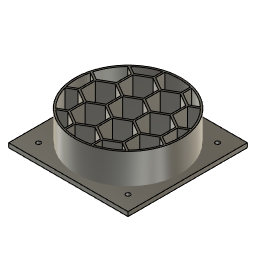
Wind Sim v6 (Autodesk Fusion 360 design; units mm, degrees)
Autodesk Fusion 360 part; units mm, degrees
(part 1 of 3)
sketch "Sketch3" plane through (0, 0, 0) normal (0, 0, 1) x (1, 0, 0)
  line L0 (-70.0229, 69.922) -> (69.9771, 69.922)
  line L1 (69.9771, 69.922) -> (69.9771, -70.078)
  line L2 (69.9771, -70.078) -> (-70.0229, -70.078)
  line L3 (-70.0229, -70.078) -> (-70.0229, 69.922)
  circle A0 centre (0, 0) radius 60
  line L4 (15, 8.6603) -> (0, 17.3205)
  line L5 (0, 17.3205) -> (-15, 8.6603)
  line L6 (-15, 8.6603) -> (-15, -8.6603)
  line L7 (-15, -8.6603) -> (0, -17.3205)
  line L8 (0, -17.3205) -> (15, -8.6603)
  line L9 (15, -8.6603) -> (15, 8.6603)
  line L10 (-15, 8.6603) -> (-15, -8.6603)
  line L11 (15, -8.6603) -> (15, 8.6603)
  line L12 (0, 17.3205) -> (-15, 8.6603)
  line L13 (15, 8.6603) -> (0, 17.3205)
  line L14 (17, 8.6603) -> (17, -8.6603)
  line L15 (17, -8.6603) -> (32, -17.3205)
  line L16 (47, -8.6603) -> (47, 8.6603)
  line L17 (47, -8.6603) -> (47, 8.6603)
  line L18 (17, 8.6603) -> (17, -8.6603)
  line L19 (47, 8.6603) -> (32, 17.3205)
  line L20 (32, -17.3205) -> (47, -8.6603)
  line L21 (32, 17.3205) -> (17, 8.6603)
  line L22 (32, 17.3205) -> (17, 8.6603)
  line L23 (47, 8.6603) -> (32, 17.3205)
  line L24 (-32, -17.3205) -> (-17, -8.6603)
  line L25 (-32, 17.3205) -> (-47, 8.6603)
  line L26 (-32, 17.3205) -> (-47, 8.6603)
  line L27 (-17, 8.6603) -> (-32, 17.3205)
  line L28 (-47, -8.6603) -> (-32, -17.3205)
  line L29 (-17, 8.6603) -> (-32, 17.3205)
  line L30 (-17, -8.6603) -> (-17, 8.6603)
  line L31 (-47, 8.6603) -> (-47, -8.6603)
  line L32 (-17, -8.6603) -> (-17, 8.6603)
  line L33 (-47, 8.6603) -> (-47, -8.6603)
  line L34 (-49, -8.6603) -> (-49, 8.6603)
  line L35 (-49, -8.6603) -> (-49, 8.6603)
  line L36 (-64, -17.3205) -> (-49, -8.6603)
  line L37 (-79, 8.6603) -> (-79, -8.6603)
  line L38 (-79, 8.6603) -> (-79, -8.6603)
  line L39 (-49, 8.6603) -> (-64, 17.3205)
  line L40 (-79, -8.6603) -> (-64, -17.3205)
  line L41 (-64, 17.3205) -> (-79, 8.6603)
  line L42 (-49, 8.6603) -> (-64, 17.3205)
  line L43 (-64, 17.3205) -> (-79, 8.6603)
  line L44 (79, -8.6603) -> (79, 8.6603)
  line L45 (49, 8.6603) -> (49, -8.6603)
  line L46 (49, 8.6603) -> (49, -8.6603)
  line L47 (79, -8.6603) -> (79, 8.6603)
  line L48 (49, -8.6603) -> (64, -17.3205)
  line L49 (64, 17.3205) -> (49, 8.6603)
  line L50 (79, 8.6603) -> (64, 17.3205)
  line L51 (64, -17.3205) -> (79, -8.6603)
  line L52 (64, 17.3205) -> (49, 8.6603)
  line L53 (79, 8.6603) -> (64, 17.3205)
  line L54 (-31, -19.3397) -> (-31, -36.6603)
  line L55 (-31, -19.3397) -> (-31, -36.6603)
  line L56 (-1, -36.6603) -> (-1, -19.3397)
  line L57 (-1, -36.6603) -> (-1, -19.3397)
  line L58 (-1, -19.3397) -> (-16, -10.6795)
  line L59 (-31, -36.6603) -> (-16, -45.3205)
  line L60 (-16, -10.6795) -> (-31, -19.3397)
  line L61 (-16, -10.6795) -> (-31, -19.3397)
  line L62 (-1, -19.3397) -> (-16, -10.6795)
  line L63 (-16, -45.3205) -> (-1, -36.6603)
  line L64 (-1, -36.6603) -> (-1, -19.3397)
  line L65 (-31, -36.6603) -> (-16, -45.3205)
  line L66 (-1, -19.3397) -> (-16, -10.6795)
  line L67 (-1, -36.6603) -> (-1, -19.3397)
  line L68 (-31, -19.3397) -> (-31, -36.6603)
  line L69 (-31, -19.3397) -> (-31, -36.6603)
  line L70 (-16, -10.6795) -> (-31, -19.3397)
  line L71 (-16, -45.3205) -> (-1, -36.6603)
  line L72 (-16, -10.6795) -> (-31, -19.3397)
  line L73 (-1, -19.3397) -> (-16, -10.6795)
  line L74 (16, -45.3205) -> (31, -36.6603)
  line L75 (31, -36.6603) -> (31, -19.3397)
  line L76 (31, -19.3397) -> (16, -10.6795)
  line L77 (16, -45.3205) -> (31, -36.6603)
  line L78 (31, -19.3397) -> (16, -10.6795)
  line L79 (1, -19.3397) -> (1, -36.6603)
  line L80 (16, -10.6795) -> (1, -19.3397)
  line L81 (1, -36.6603) -> (16, -45.3205)
  line L82 (1, -19.3397) -> (1, -36.6603)
  line L83 (1, -19.3397) -> (1, -36.6603)
  line L84 (16, -10.6795) -> (1, -19.3397)
  line L85 (31, -36.6603) -> (31, -19.3397)
  line L86 (31, -36.6603) -> (31, -19.3397)
  line L87 (16, -10.6795) -> (1, -19.3397)
  line L88 (1, -19.3397) -> (1, -36.6603)
  line L89 (31, -19.3397) -> (16, -10.6795)
  line L90 (31, -19.3397) -> (16, -10.6795)
  line L91 (31, -36.6603) -> (31, -19.3397)
  line L92 (1, -36.6603) -> (16, -45.3205)
  line L93 (16, -10.6795) -> (1, -19.3397)
  line L94 (-48, -10.6795) -> (-63, -19.3397)
  line L95 (-63, -36.6603) -> (-48, -45.3205)
  line L96 (-48, -10.6795) -> (-63, -19.3397)
  line L97 (-48, -10.6795) -> (-63, -19.3397)
  line L98 (-63, -36.6603) -> (-48, -45.3205)
  line L99 (-33, -19.3397) -> (-48, -10.6795)
  line L100 (-48, -10.6795) -> (-63, -19.3397)
  line L101 (-33, -19.3397) -> (-48, -10.6795)
  line L102 (-63, -19.3397) -> (-63, -36.6603)
  line L103 (-63, -19.3397) -> (-63, -36.6603)
  line L104 (-33, -36.6603) -> (-33, -19.3397)
  line L105 (-33, -36.6603) -> (-33, -19.3397)
  line L106 (-33, -19.3397) -> (-48, -10.6795)
  line L107 (-63, -19.3397) -> (-63, -36.6603)
  line L108 (-33, -36.6603) -> (-33, -19.3397)
  line L109 (-63, -19.3397) -> (-63, -36.6603)
  line L110 (-48, -45.3205) -> (-33, -36.6603)
  line L111 (-33, -36.6603) -> (-33, -19.3397)
  line L112 (-33, -19.3397) -> (-48, -10.6795)
  line L113 (-48, -45.3205) -> (-33, -36.6603)
  line L114 (33, -19.3397) -> (33, -36.6603)
  line L115 (48, -10.6795) -> (33, -19.3397)
  line L116 (63, -19.3397) -> (48, -10.6795)
  line L117 (63, -36.6603) -> (63, -19.3397)
  line L118 (48, -45.3205) -> (63, -36.6603)
  line L119 (33, -36.6603) -> (48, -45.3205)
  line L120 (-47, -47.3397) -> (-47, -64.6603)
  line L121 (-49, -64.6603) -> (-49, -47.3397)
  line L122 (-17, -64.6603) -> (-17, -47.3397)
  line L123 (47, -64.6603) -> (47, -47.3397)
  line L124 (17, -47.3397) -> (17, -64.6603)
  line L125 (-15, -64.6603) -> (0, -73.3205)
  line L126 (-1, -75.3397) -> (-16, -66.6795)
  line L127 (79, -64.6603) -> (79, -47.3397)
  line L128 (49, -47.3397) -> (49, -64.6603)
  line L129 (-1, -75.3397) -> (-16, -66.6795)
  line L130 (-15, -47.3397) -> (-15, -64.6603)
  line L131 (49, -47.3397) -> (49, -64.6603)
  line L132 (47, -64.6603) -> (47, -47.3397)
  line L133 (-15, -47.3397) -> (-15, -64.6603)
  line L134 (-47, -47.3397) -> (-47, -64.6603)
  line L135 (-1, -75.3397) -> (-16, -66.6795)
  line L136 (15, -64.6603) -> (15, -47.3397)
  line L137 (-17, -47.3397) -> (-32, -38.6795)
  line L138 (-64, -73.3205) -> (-49, -64.6603)
  line L139 (31, -75.3397) -> (16, -66.6795)
  line L140 (-48, -66.6795) -> (-63, -75.3397)
  line L141 (-17, -47.3397) -> (-32, -38.6795)
  line L142 (64, -38.6795) -> (49, -47.3397)
  line L143 (-48, -66.6795) -> (-63, -75.3397)
  line L144 (15, -47.3397) -> (0, -38.6795)
  line L145 (-33, -75.3397) -> (-48, -66.6795)
  line L146 (16, -66.6795) -> (1, -75.3397)
  line L147 (-32, -38.6795) -> (-47, -47.3397)
  line L148 (-33, -75.3397) -> (-48, -66.6795)
  line L149 (-47, -64.6603) -> (-32, -73.3205)
  line L150 (0, -38.6795) -> (-15, -47.3397)
  line L151 (32, -38.6795) -> (17, -47.3397)
  line L152 (-49, -47.3397) -> (-64, -38.6795)
  line L153 (64, -38.6795) -> (49, -47.3397)
  line L154 (-48, -66.6795) -> (-63, -75.3397)
  line L155 (47, -47.3397) -> (32, -38.6795)
  line L156 (-32, -38.6795) -> (-47, -47.3397)
  line L157 (-33, -75.3397) -> (-48, -66.6795)
  line L158 (-16, -66.6795) -> (-31, -75.3397)
  line L159 (79, -47.3397) -> (64, -38.6795)
  line L160 (15, -47.3397) -> (0, -38.6795)
  line L161 (-33, -75.3397) -> (-48, -66.6795)
  line L162 (32, -38.6795) -> (17, -47.3397)
  line L163 (-48, -66.6795) -> (-63, -75.3397)
  line L164 (-49, -47.3397) -> (-64, -38.6795)
  line L165 (-49, -64.6603) -> (-49, -47.3397)
  line L166 (-1, -75.3397) -> (-16, -66.6795)
  line L167 (79, -64.6603) -> (79, -47.3397)
  line L168 (-17, -64.6603) -> (-17, -47.3397)
  line L169 (15, -64.6603) -> (15, -47.3397)
  line L170 (0, -73.3205) -> (15, -64.6603)
  line L171 (-32, -73.3205) -> (-17, -64.6603)
  line L172 (0, -38.6795) -> (-15, -47.3397)
  line L173 (-16, -66.6795) -> (-31, -75.3397)
  line L174 (-16, -66.6795) -> (-31, -75.3397)
  line L175 (-16, -66.6795) -> (-31, -75.3397)
  line L176 (17, -47.3397) -> (17, -64.6603)
  line L177 (64, -73.3205) -> (79, -64.6603)
  line L178 (31, -75.3397) -> (16, -66.6795)
  line L179 (32, -73.3205) -> (47, -64.6603)
  line L180 (31, -75.3397) -> (16, -66.6795)
  line L181 (47, -47.3397) -> (32, -38.6795)
  line L182 (31, -75.3397) -> (16, -66.6795)
  line L183 (48, -66.6795) -> (33, -75.3397)
  line L184 (16, -66.6795) -> (1, -75.3397)
  line L185 (16, -66.6795) -> (1, -75.3397)
  line L186 (17, -64.6603) -> (32, -73.3205)
  line L187 (79, -47.3397) -> (64, -38.6795)
  line L188 (16, -66.6795) -> (1, -75.3397)
  line L189 (49, -64.6603) -> (64, -73.3205)
  line L190 (63, -75.3397) -> (48, -66.6795)
  line L191 (-31, -36.6603) -> (-16, -45.3205)
  line L192 (-16, -66.6795) -> (-31, -75.3397)
  line L193 (33, -36.6603) -> (48, -45.3205)
  line L194 (-63, -19.3397) -> (-63, -36.6603)
  line L195 (-16, -45.3205) -> (-1, -36.6603)
  line L196 (-1, -19.3397) -> (-16, -10.6795)
  line L197 (-1, -36.6603) -> (-1, -19.3397)
  line L198 (-1, -19.3397) -> (-16, -10.6795)
  line L199 (-32, -38.6795) -> (-47, -47.3397)
  line L200 (-1, -36.6603) -> (-1, -19.3397)
  line L201 (49, -8.6603) -> (64, -17.3205)
  line L202 (31, -36.6603) -> (31, -19.3397)
  line L203 (-33, -36.6603) -> (-33, -19.3397)
  line L204 (48, -66.6795) -> (33, -75.3397)
  line L205 (-48, -45.3205) -> (-33, -36.6603)
  line L206 (16, -45.3205) -> (31, -36.6603)
  line L207 (1, -36.6603) -> (16, -45.3205)
  line L208 (31, -36.6603) -> (31, -19.3397)
  line L209 (-16, -66.6795) -> (-31, -75.3397)
  line L210 (-63, -36.6603) -> (-48, -45.3205)
  line L211 (16, -10.6795) -> (1, -19.3397)
  line L212 (31, -19.3397) -> (16, -10.6795)
  line L213 (-1, -19.3397) -> (-16, -10.6795)
  line L214 (63, -75.3397) -> (48, -66.6795)
  line L215 (63, -36.6603) -> (63, -19.3397)
  line L216 (31, -36.6603) -> (31, -19.3397)
  line L217 (-32, -38.6795) -> (-47, -47.3397)
  line L218 (31, -36.6603) -> (31, -19.3397)
  line L219 (1, -19.3397) -> (1, -36.6603)
  line L220 (16, -45.3205) -> (31, -36.6603)
  line L221 (-16, -66.6795) -> (-31, -75.3397)
  line L222 (1, -19.3397) -> (1, -36.6603)
  line L223 (-17, -47.3397) -> (-32, -38.6795)
  line L224 (-32, -73.3205) -> (-17, -64.6603)
  line L225 (-17, -47.3397) -> (-32, -38.6795)
  line L226 (-16, -66.6795) -> (-31, -75.3397)
  line L227 (31, -19.3397) -> (16, -10.6795)
  line L228 (48, -10.6795) -> (33, -19.3397)
  line L229 (-49, -47.3397) -> (-64, -38.6795)
  line L230 (1, -36.6603) -> (16, -45.3205)
  line L231 (-49, -47.3397) -> (-64, -38.6795)
  line L232 (-1, -19.3397) -> (-16, -10.6795)
  line L233 (-79, -8.6603) -> (-64, -17.3205)
  line L234 (48, -45.3205) -> (63, -36.6603)
  line L235 (-15, -8.6603) -> (0, -17.3205)
  line L236 (0, -17.3205) -> (15, -8.6603)
  line L237 (15, -47.3397) -> (0, -38.6795)
  line L238 (-16, -10.6795) -> (-31, -19.3397)
  line L239 (1, -19.3397) -> (1, -36.6603)
  line L240 (-16, -10.6795) -> (-31, -19.3397)
  line L241 (-32, -17.3205) -> (-17, -8.6603)
  line L242 (1, -19.3397) -> (1, -36.6603)
  line L243 (-1, -36.6603) -> (-1, -19.3397)
  line L244 (-1, -36.6603) -> (-1, -19.3397)
  line L245 (-15, -47.3397) -> (-15, -64.6603)
  line L246 (0, -73.3205) -> (15, -64.6603)
  line L247 (15, -47.3397) -> (0, -38.6795)
  line L248 (33, -19.3397) -> (33, -36.6603)
  line L249 (69.9771, -70.078) -> (-70.0229, -70.078)
  line L250 (-16, -10.6795) -> (-31, -19.3397)
  line L251 (-16, -10.6795) -> (-31, -19.3397)
  line L252 (-31, -36.6603) -> (-16, -45.3205)
  line L253 (-16, -45.3205) -> (-1, -36.6603)
  line L254 (-15, -47.3397) -> (-15, -64.6603)
  line L255 (-15, -64.6603) -> (0, -73.3205)
  line L256 (0, -38.6795) -> (-15, -47.3397)
  line L257 (-1, -75.3397) -> (-16, -66.6795)
  line L258 (-1, -75.3397) -> (-16, -66.6795)
  line L259 (-1, -75.3397) -> (-16, -66.6795)
  line L260 (64, -38.6795) -> (49, -47.3397)
  line L261 (31, -75.3397) -> (16, -66.6795)
  line L262 (-33, -75.3397) -> (-48, -66.6795)
  line L263 (49, -47.3397) -> (49, -64.6603)
  line L264 (17, -64.6603) -> (32, -73.3205)
  line L265 (49, -64.6603) -> (64, -73.3205)
  line L266 (64, -38.6795) -> (49, -47.3397)
  line L267 (47, -64.6603) -> (47, -47.3397)
  line L268 (-64, -73.3205) -> (-49, -64.6603)
  line L269 (-31, -19.3397) -> (-31, -36.6603)
  line L270 (47, -47.3397) -> (32, -38.6795)
  line L271 (-33, -36.6603) -> (-33, -19.3397)
  line L272 (-48, -66.6795) -> (-63, -75.3397)
  line L273 (-33, -75.3397) -> (-48, -66.6795)
  line L274 (49, -47.3397) -> (49, -64.6603)
  line L275 (16, -66.6795) -> (1, -75.3397)
  line L276 (32, -38.6795) -> (17, -47.3397)
  line L277 (79, -47.3397) -> (64, -38.6795)
  line L278 (16, -66.6795) -> (1, -75.3397)
  line L279 (-49, -64.6603) -> (-49, -47.3397)
  line L280 (47, -47.3397) -> (32, -38.6795)
  line L281 (-33, -36.6603) -> (-33, -19.3397)
  line L282 (31, -75.3397) -> (16, -66.6795)
  line L283 (-31, -19.3397) -> (-31, -36.6603)
  line L284 (-48, -10.6795) -> (-63, -19.3397)
  line L285 (47, -64.6603) -> (47, -47.3397)
  line L286 (16, -66.6795) -> (1, -75.3397)
  line L287 (-48, -10.6795) -> (-63, -19.3397)
  line L288 (-33, -19.3397) -> (-48, -10.6795)
  line L289 (16, -66.6795) -> (1, -75.3397)
  line L290 (31, -19.3397) -> (16, -10.6795)
  line L291 (-31, -19.3397) -> (-31, -36.6603)
  line L292 (-48, -10.6795) -> (-63, -19.3397)
  line L293 (-47, -64.6603) -> (-32, -73.3205)
  line L294 (-33, -75.3397) -> (-48, -66.6795)
  line L295 (-33, -19.3397) -> (-48, -10.6795)
  line L296 (-63, -36.6603) -> (-48, -45.3205)
  line L297 (64, -73.3205) -> (79, -64.6603)
  line L298 (16, -10.6795) -> (1, -19.3397)
  line L299 (-49, -64.6603) -> (-49, -47.3397)
  line L300 (-48, -10.6795) -> (-63, -19.3397)
  line L301 (31, -19.3397) -> (16, -10.6795)
  line L302 (-63, -19.3397) -> (-63, -36.6603)
  line L303 (15, -64.6603) -> (15, -47.3397)
  line L304 (17, -47.3397) -> (17, -64.6603)
  line L305 (79, -64.6603) -> (79, -47.3397)
  line L306 (16, -10.6795) -> (1, -19.3397)
  line L307 (16, -10.6795) -> (1, -19.3397)
  line L308 (-33, -36.6603) -> (-33, -19.3397)
  line L309 (-64, -17.3205) -> (-49, -8.6603)
  line L310 (32, -17.3205) -> (47, -8.6603)
  line L311 (-33, -75.3397) -> (-48, -66.6795)
  line L312 (-33, -19.3397) -> (-48, -10.6795)
  line L313 (-47, -8.6603) -> (-32, -17.3205)
  line L314 (-31, -19.3397) -> (-31, -36.6603)
  line L315 (17, -8.6603) -> (32, -17.3205)
  line L316 (31, -75.3397) -> (16, -66.6795)
  line L317 (64, -17.3205) -> (79, -8.6603)
  line L318 (-63, -19.3397) -> (-63, -36.6603)
  line L319 (-48, -66.6795) -> (-63, -75.3397)
  line L320 (-63, -19.3397) -> (-63, -36.6603)
  line L321 (15, -64.6603) -> (15, -47.3397)
  line L322 (32, -73.3205) -> (47, -64.6603)
  line L323 (-47, -47.3397) -> (-47, -64.6603)
  line L324 (-47, -47.3397) -> (-47, -64.6603)
  line L325 (79, -47.3397) -> (64, -38.6795)
  line L326 (-33, -19.3397) -> (-48, -10.6795)
  line L327 (79, -64.6603) -> (79, -47.3397)
  line L328 (-48, -66.6795) -> (-63, -75.3397)
  line L329 (31, -75.3397) -> (16, -66.6795)
  line L330 (-48, -66.6795) -> (-63, -75.3397)
  line L331 (32, -38.6795) -> (17, -47.3397)
  line L332 (-48, -45.3205) -> (-33, -36.6603)
  line L333 (17, -47.3397) -> (17, -64.6603)
  line L334 (63, -19.3397) -> (48, -10.6795)
  line L335 (-17, -64.6603) -> (-17, -47.3397)
  line L336 (-1, -75.3397) -> (-16, -66.6795)
  line L337 (0, -38.6795) -> (-15, -47.3397)
  line L338 (-17, -64.6603) -> (-17, -47.3397)
  line L339 (-1, -19.3397) -> (-16, -10.6795)
  line L340 (-1, -36.6603) -> (-1, -19.3397)
  line L341 (-1, -36.6603) -> (-1, -19.3397)
  line L342 (-1, -19.3397) -> (-16, -10.6795)
  line L343 (-1, -19.3397) -> (-16, -10.6795)
  line L344 (-1, -36.6603) -> (-1, -19.3397)
  line L345 (15, -47.3397) -> (0, -38.6795)
  line L346 (-16, -45.3205) -> (-1, -36.6603)
  line L347 (0, -17.3205) -> (15, -8.6603)
  line L348 (15, -47.3397) -> (0, -38.6795)
  line L349 (15, -47.3397) -> (0, -38.6795)
  line L350 (15, -47.3397) -> (0, -38.6795)
  line L351 (0, -17.3205) -> (15, -8.6603)
  line L352 (-17, -47.3397) -> (-32, -38.6795)
  line L353 (-31, -36.6603) -> (-16, -45.3205)
  line L354 (-16, -45.3205) -> (-1, -36.6603)
  line L355 (-16, -10.6795) -> (-31, -19.3397)
  line L356 (31, -36.6603) -> (31, -19.3397)
  line L357 (-17, -47.3397) -> (-32, -38.6795)
  line L358 (-16, -10.6795) -> (-31, -19.3397)
  line L359 (0, -38.6795) -> (-15, -47.3397)
  line L360 (1, -19.3397) -> (1, -36.6603)
  line L361 (-15, -8.6603) -> (0, -17.3205)
  line L362 (0, -38.6795) -> (-15, -47.3397)
  line L363 (-1, -19.3397) -> (-16, -10.6795)
  line L364 (-1, -19.3397) -> (-16, -10.6795)
  line L365 (-1, -36.6603) -> (-1, -19.3397)
  line L366 (0, -38.6795) -> (-15, -47.3397)
  line L367 (-16, -45.3205) -> (-1, -36.6603)
  line L368 (-16, -45.3205) -> (-1, -36.6603)
  line L369 (-1, -36.6603) -> (-1, -19.3397)
  line L370 (0, -38.6795) -> (-15, -47.3397)
  line L371 (-1, -19.3397) -> (-16, -10.6795)
  line L372 (-1, -19.3397) -> (-16, -10.6795)
  line L373 (-1, -36.6603) -> (-1, -19.3397)
  line L374 (-15, -8.6603) -> (0, -17.3205)
  line L375 (-1, -36.6603) -> (-1, -19.3397)
  line L376 (-32, -17.3205) -> (-17, -8.6603)
  line L377 (-16, -10.6795) -> (-31, -19.3397)
  line L378 (1, -19.3397) -> (1, -36.6603)
  line L379 (-16, -10.6795) -> (-31, -19.3397)
  line L380 (-1, -19.3397) -> (-16, -10.6795)
  line L381 (1, -19.3397) -> (1, -36.6603)
  line L382 (-48, -45.3205) -> (-33, -36.6603)
  line L383 (-17, -64.6603) -> (-17, -47.3397)
  line L384 (-32, -38.6795) -> (-47, -47.3397)
  line L385 (-49, -47.3397) -> (-64, -38.6795)
  line L386 (-63, -36.6603) -> (-48, -45.3205)
  line L387 (63, -36.6603) -> (63, -19.3397)
  line L388 (-15, -47.3397) -> (-15, -64.6603)
  line L389 (-31, -36.6603) -> (-16, -45.3205)
  line L390 (-32, -38.6795) -> (-47, -47.3397)
  line L391 (64, -17.3205) -> (79, -8.6603)
  line L392 (33, -19.3397) -> (33, -36.6603)
  line L393 (31, -36.6603) -> (31, -19.3397)
  line L394 (63, -36.6603) -> (63, -19.3397)
  line L395 (-15, -47.3397) -> (-15, -64.6603)
  line L396 (32, -38.6795) -> (17, -47.3397)
  line L397 (16, -10.6795) -> (1, -19.3397)
  line L398 (1, -19.3397) -> (1, -36.6603)
  line L399 (-63, -36.6603) -> (-48, -45.3205)
  line L400 (-49, -47.3397) -> (-64, -38.6795)
  line L401 (31, -36.6603) -> (31, -19.3397)
  line L402 (31, -36.6603) -> (31, -19.3397)
  line L403 (-31, -36.6603) -> (-16, -45.3205)
  line L404 (-48, -45.3205) -> (-33, -36.6603)
  line L405 (-48, -45.3205) -> (-33, -36.6603)
  line L406 (-63, -36.6603) -> (-48, -45.3205)
  line L407 (-32, -38.6795) -> (-47, -47.3397)
  line L408 (16, -10.6795) -> (1, -19.3397)
  line L409 (33, -19.3397) -> (33, -36.6603)
  line L410 (-32, -17.3205) -> (-17, -8.6603)
  line L411 (-16, -10.6795) -> (-31, -19.3397)
  line L412 (-17, -47.3397) -> (-32, -38.6795)
  line L413 (1, -19.3397) -> (1, -36.6603)
  line L414 (31, -36.6603) -> (31, -19.3397)
  line L415 (-17, -64.6603) -> (-17, -47.3397)
  line L416 (31, -36.6603) -> (31, -19.3397)
  line L417 (-16, -10.6795) -> (-31, -19.3397)
  line L418 (-15, -47.3397) -> (-15, -64.6603)
  line L419 (-63, -36.6603) -> (-48, -45.3205)
  line L420 (-17, -64.6603) -> (-17, -47.3397)
  line L421 (31, -19.3397) -> (16, -10.6795)
  line L422 (-49, -47.3397) -> (-64, -38.6795)
  line L423 (17, -8.6603) -> (32, -17.3205)
  line L424 (-31, -36.6603) -> (-16, -45.3205)
  line L425 (31, -36.6603) -> (31, -19.3397)
  line L426 (-48, -45.3205) -> (-33, -36.6603)
  line L427 (1, -19.3397) -> (1, -36.6603)
  line L428 (-17, -64.6603) -> (-17, -47.3397)
  line L429 (-32, -38.6795) -> (-47, -47.3397)
  line L430 (32, -38.6795) -> (17, -47.3397)
  line L431 (-1, -36.6603) -> (-1, -19.3397)
  line L432 (1, -19.3397) -> (1, -36.6603)
  line L433 (-16, -10.6795) -> (-31, -19.3397)
  line L434 (-17, -47.3397) -> (-32, -38.6795)
  line L435 (-16, -10.6795) -> (-31, -19.3397)
  line L436 (31, -36.6603) -> (31, -19.3397)
  line L437 (-15, -47.3397) -> (-15, -64.6603)
  line L438 (-49, -47.3397) -> (-64, -38.6795)
  line L439 (1, -19.3397) -> (1, -36.6603)
  line L440 (-48, -10.6795) -> (-63, -19.3397)
  line L441 (1, -36.6603) -> (16, -45.3205)
  line L442 (47, -64.6603) -> (47, -47.3397)
  line L443 (48, -10.6795) -> (33, -19.3397)
  line L444 (63, -19.3397) -> (48, -10.6795)
  line L445 (-48, -10.6795) -> (-63, -19.3397)
  line L446 (49, -8.6603) -> (64, -17.3205)
  line L447 (1, -36.6603) -> (16, -45.3205)
  line L448 (17, -47.3397) -> (17, -64.6603)
  line L449 (-48, -10.6795) -> (-63, -19.3397)
  line L450 (-48, -10.6795) -> (-63, -19.3397)
  line L451 (16, -10.6795) -> (1, -19.3397)
  line L452 (-49, -64.6603) -> (-49, -47.3397)
  line L453 (-47, -47.3397) -> (-47, -64.6603)
  line L454 (16, -10.6795) -> (1, -19.3397)
  line L455 (33, -36.6603) -> (48, -45.3205)
  line L456 (48, -10.6795) -> (33, -19.3397)
  line L457 (-48, -10.6795) -> (-63, -19.3397)
  line L458 (-49, -64.6603) -> (-49, -47.3397)
  line L459 (32, -17.3205) -> (47, -8.6603)
  line L460 (-33, -19.3397) -> (-48, -10.6795)
  line L461 (-48, -10.6795) -> (-63, -19.3397)
  line L462 (64, -17.3205) -> (79, -8.6603)
  line L463 (32, -38.6795) -> (17, -47.3397)
  line L464 (47, -47.3397) -> (32, -38.6795)
  line L465 (31, -19.3397) -> (16, -10.6795)
  line L466 (-33, -19.3397) -> (-48, -10.6795)
  line L467 (79, -47.3397) -> (64, -38.6795)
  line L468 (15, -64.6603) -> (15, -47.3397)
  line L469 (-48, -10.6795) -> (-63, -19.3397)
  line L470 (31, -19.3397) -> (16, -10.6795)
  line L471 (47, -64.6603) -> (47, -47.3397)
  line L472 (-33, -19.3397) -> (-48, -10.6795)
  line L473 (16, -10.6795) -> (1, -19.3397)
  line L474 (16, -10.6795) -> (1, -19.3397)
  line L475 (-33, -19.3397) -> (-48, -10.6795)
  line L476 (-33, -19.3397) -> (-48, -10.6795)
  line L477 (-33, -19.3397) -> (-48, -10.6795)
  line L478 (31, -19.3397) -> (16, -10.6795)
  line L479 (-47, -47.3397) -> (-47, -64.6603)
  line L480 (-48, -10.6795) -> (-63, -19.3397)
  line L481 (31, -19.3397) -> (16, -10.6795)
  line L482 (49, -8.6603) -> (64, -17.3205)
  line L483 (79, -64.6603) -> (79, -47.3397)
  line L484 (64, -38.6795) -> (49, -47.3397)
  line L485 (48, -45.3205) -> (63, -36.6603)
  line L486 (-49, -64.6603) -> (-49, -47.3397)
  line L487 (-33, -19.3397) -> (-48, -10.6795)
  line L488 (-33, -19.3397) -> (-48, -10.6795)
  line L489 (-47, -8.6603) -> (-32, -17.3205)
  line L490 (33, -36.6603) -> (48, -45.3205)
  line L491 (16, -45.3205) -> (31, -36.6603)
  line L492 (79, -47.3397) -> (64, -38.6795)
  line L493 (-63, -19.3397) -> (-63, -36.6603)
  line L494 (49, -47.3397) -> (49, -64.6603)
  line L495 (15, -64.6603) -> (15, -47.3397)
  line L496 (-79, -8.6603) -> (-64, -17.3205)
  line L497 (-64, -17.3205) -> (-49, -8.6603)
  line L498 (64, -38.6795) -> (49, -47.3397)
  line L499 (47, -64.6603) -> (47, -47.3397)
  line L500 (15, -64.6603) -> (15, -47.3397)
  line L501 (49, -47.3397) -> (49, -64.6603)
  line L502 (47, -47.3397) -> (32, -38.6795)
  line L503 (79, -47.3397) -> (64, -38.6795)
  line L504 (-33, -36.6603) -> (-33, -19.3397)
  line L505 (1, -36.6603) -> (16, -45.3205)
  line L506 (79, -64.6603) -> (79, -47.3397)
  line L507 (17, -47.3397) -> (17, -64.6603)
  line L508 (64, -38.6795) -> (49, -47.3397)
  line L509 (-33, -36.6603) -> (-33, -19.3397)
  line L510 (-33, -36.6603) -> (-33, -19.3397)
  line L511 (16, -45.3205) -> (31, -36.6603)
  line L512 (47, -64.6603) -> (47, -47.3397)
  line L513 (-63, -19.3397) -> (-63, -36.6603)
  line L514 (-79, -8.6603) -> (-64, -17.3205)
  line L515 (-47, -47.3397) -> (-47, -64.6603)
  line L516 (1, -36.6603) -> (16, -45.3205)
  line L517 (79, -47.3397) -> (64, -38.6795)
  line L518 (-64, -17.3205) -> (-49, -8.6603)
  line L519 (-33, -36.6603) -> (-33, -19.3397)
  line L520 (17, -47.3397) -> (17, -64.6603)
  line L521 (16, -10.6795) -> (1, -19.3397)
  line L522 (-31, -19.3397) -> (-31, -36.6603)
  line L523 (16, -45.3205) -> (31, -36.6603)
  line L524 (-63, -19.3397) -> (-63, -36.6603)
  line L525 (-63, -19.3397) -> (-63, -36.6603)
  line L526 (-31, -19.3397) -> (-31, -36.6603)
  line L527 (-47, -47.3397) -> (-47, -64.6603)
  line L528 (17, -8.6603) -> (32, -17.3205)
  line L529 (79, -64.6603) -> (79, -47.3397)
  line L530 (16, -45.3205) -> (31, -36.6603)
  line L531 (-33, -36.6603) -> (-33, -19.3397)
  line L532 (64, -38.6795) -> (49, -47.3397)
  line L533 (-63, -19.3397) -> (-63, -36.6603)
  line L534 (32, -38.6795) -> (17, -47.3397)
  line L535 (31, -19.3397) -> (16, -10.6795)
  line L536 (63, -19.3397) -> (48, -10.6795)
  line L537 (-31, -19.3397) -> (-31, -36.6603)
  line L538 (31, -19.3397) -> (16, -10.6795)
  line L539 (-47, -8.6603) -> (-32, -17.3205)
  line L540 (-31, -19.3397) -> (-31, -36.6603)
  line L541 (32, -17.3205) -> (47, -8.6603)
  line L542 (-33, -36.6603) -> (-33, -19.3397)
  line L543 (-31, -19.3397) -> (-31, -36.6603)
  line L544 (-31, -19.3397) -> (-31, -36.6603)
  line L545 (-31, -19.3397) -> (-31, -36.6603)
  line L546 (79, -64.6603) -> (79, -47.3397)
  line L547 (16, -10.6795) -> (1, -19.3397)
  line L548 (-63, -19.3397) -> (-63, -36.6603)
  line L549 (-33, -36.6603) -> (-33, -19.3397)
  line L550 (-63, -19.3397) -> (-63, -36.6603)
  line L551 (-33, -36.6603) -> (-33, -19.3397)
  line L552 (47, -47.3397) -> (32, -38.6795)
  line L553 (49, -47.3397) -> (49, -64.6603)
  line L554 (47, -47.3397) -> (32, -38.6795)
  line L555 (48, -45.3205) -> (63, -36.6603)
  line L556 (49, -47.3397) -> (49, -64.6603)
  line L557 (-31, -19.3397) -> (-31, -36.6603)
  line L558 (15, -64.6603) -> (15, -47.3397)
  line L559 (31, -19.3397) -> (16, -10.6795)
  line L560 (17, -47.3397) -> (17, -64.6603)
  line L561 (-49, -64.6603) -> (-49, -47.3397)
  line L562 (-63, -19.3397) -> (-63, -36.6603)
  line L563 (-47, -64.6603) -> (-32, -73.3205)
  line L564 (-32, -73.3205) -> (-17, -64.6603)
  line L565 (-15, -64.6603) -> (0, -73.3205)
  line L566 (0, -73.3205) -> (15, -64.6603)
  line L567 (17, -64.6603) -> (32, -73.3205)
  line L568 (32, -73.3205) -> (47, -64.6603)
  line L569 (49, -64.6603) -> (64, -73.3205)
  line L570 (64, -73.3205) -> (79, -64.6603)
  line L571 (-64, -73.3205) -> (-49, -64.6603)
  line L572 (63, 19.3397) -> (63, 36.6603)
  line L573 (1, 36.6603) -> (1, 19.3397)
  line L574 (63, 19.3397) -> (63, 36.6603)
  line L575 (31, 19.3397) -> (31, 36.6603)
  line L576 (1, 36.6603) -> (1, 19.3397)
  line L577 (31, 19.3397) -> (31, 36.6603)
  line L578 (31, 19.3397) -> (31, 36.6603)
  line L579 (31, 19.3397) -> (31, 36.6603)
  line L580 (1, 36.6603) -> (1, 19.3397)
  line L581 (1, 36.6603) -> (1, 19.3397)
  line L582 (31, 19.3397) -> (31, 36.6603)
  line L583 (1, 36.6603) -> (1, 19.3397)
  line L584 (33, 36.6603) -> (33, 19.3397)
  line L585 (-31, 36.6603) -> (-31, 19.3397)
  line L586 (31, 19.3397) -> (31, 36.6603)
  line L587 (-63, 36.6603) -> (-63, 19.3397)
  line L588 (-63, 36.6603) -> (-63, 19.3397)
  line L589 (-33, 19.3397) -> (-33, 36.6603)
  line L590 (-31, 36.6603) -> (-31, 19.3397)
  line L591 (-33, 19.3397) -> (-33, 36.6603)
  line L592 (-33, 19.3397) -> (-33, 36.6603)
  line L593 (-63, 36.6603) -> (-63, 19.3397)
  line L594 (31, 19.3397) -> (31, 36.6603)
  line L595 (33, 36.6603) -> (33, 19.3397)
  line L596 (-31, 36.6603) -> (-31, 19.3397)
  line L597 (-1, 19.3397) -> (-1, 36.6603)
  line L598 (-1, 19.3397) -> (-1, 36.6603)
  line L599 (-1, 19.3397) -> (-1, 36.6603)
  line L600 (1, 36.6603) -> (1, 19.3397)
  line L601 (-1, 19.3397) -> (-1, 36.6603)
  line L602 (-31, 36.6603) -> (-31, 19.3397)
  line L603 (-31, 36.6603) -> (-31, 19.3397)
  line L604 (-63, 36.6603) -> (-63, 19.3397)
  line L605 (-63, 36.6603) -> (-63, 19.3397)
  line L606 (-1, 19.3397) -> (-1, 36.6603)
  line L607 (-63, 36.6603) -> (-63, 19.3397)
  line L608 (-1, 19.3397) -> (-1, 36.6603)
  line L609 (-63, 36.6603) -> (-63, 19.3397)
  line L610 (-63, 36.6603) -> (-63, 19.3397)
  line L611 (-63, 36.6603) -> (-63, 19.3397)
  line L612 (-33, 19.3397) -> (-33, 36.6603)
  line L613 (-63, 36.6603) -> (-63, 19.3397)
  line L614 (1, 36.6603) -> (1, 19.3397)
  line L615 (-1, 19.3397) -> (-1, 36.6603)
  line L616 (31, 19.3397) -> (31, 36.6603)
  line L617 (-1, 19.3397) -> (-1, 36.6603)
  line L618 (-1, 19.3397) -> (-1, 36.6603)
  line L619 (-1, 19.3397) -> (-1, 36.6603)
  line L620 (-31, 36.6603) -> (-31, 19.3397)
  line L621 (-63, 36.6603) -> (-63, 19.3397)
  line L622 (-31, 36.6603) -> (-31, 19.3397)
  line L623 (-1, 19.3397) -> (-1, 36.6603)
  line L624 (-1, 19.3397) -> (-1, 36.6603)
  line L625 (-1, 19.3397) -> (-1, 36.6603)
  line L626 (-31, 36.6603) -> (-31, 19.3397)
  line L627 (31, 19.3397) -> (31, 36.6603)
  line L628 (1, 36.6603) -> (1, 19.3397)
  line L629 (-31, 36.6603) -> (-31, 19.3397)
  line L630 (-63, 36.6603) -> (-63, 19.3397)
  line L631 (-33, 19.3397) -> (-33, 36.6603)
  line L632 (-33, 19.3397) -> (-33, 36.6603)
  line L633 (-31, 36.6603) -> (-31, 19.3397)
  line L634 (-33, 19.3397) -> (-33, 36.6603)
  line L635 (-33, 19.3397) -> (-33, 36.6603)
  line L636 (-63, 36.6603) -> (-63, 19.3397)
  line L637 (1, 36.6603) -> (1, 19.3397)
  line L638 (1, 36.6603) -> (1, 19.3397)
  line L639 (1, 36.6603) -> (1, 19.3397)
  line L640 (1, 36.6603) -> (1, 19.3397)
  line L641 (-1, 19.3397) -> (-1, 36.6603)
  line L642 (1, 36.6603) -> (1, 19.3397)
  line L643 (63, 19.3397) -> (63, 36.6603)
  line L644 (-1, 19.3397) -> (-1, 36.6603)
  line L645 (1, 36.6603) -> (1, 19.3397)
  line L646 (33, 36.6603) -> (33, 19.3397)
  line L647 (1, 36.6603) -> (1, 19.3397)
  line L648 (31, 19.3397) -> (31, 36.6603)
  line L649 (31, 19.3397) -> (31, 36.6603)
  line L650 (-1, 19.3397) -> (-1, 36.6603)
  line L651 (1, 36.6603) -> (1, 19.3397)
  line L652 (31, 19.3397) -> (31, 36.6603)
  line L653 (31, 19.3397) -> (31, 36.6603)
  line L654 (33, 36.6603) -> (33, 19.3397)
  line L655 (31, 19.3397) -> (31, 36.6603)
  line L656 (63, 19.3397) -> (63, 36.6603)
  line L657 (31, 19.3397) -> (31, 36.6603)
  line L658 (31, 19.3397) -> (31, 36.6603)
  line L659 (-31, 36.6603) -> (-31, 19.3397)
  line L660 (-63, 36.6603) -> (-63, 19.3397)
  line L661 (-33, 19.3397) -> (-33, 36.6603)
  line L662 (-33, 19.3397) -> (-33, 36.6603)
  line L663 (-33, 19.3397) -> (-33, 36.6603)
  line L664 (-63, 36.6603) -> (-63, 19.3397)
  line L665 (-31, 36.6603) -> (-31, 19.3397)
  line L666 (-31, 36.6603) -> (-31, 19.3397)
  line L667 (-31, 36.6603) -> (-31, 19.3397)
  line L668 (-31, 36.6603) -> (-31, 19.3397)
  line L669 (-33, 19.3397) -> (-33, 36.6603)
  line L670 (-33, 19.3397) -> (-33, 36.6603)
  line L671 (-33, 19.3397) -> (-33, 36.6603)
  line L672 (-31, 36.6603) -> (-31, 19.3397)
  line L673 (-63, 36.6603) -> (-63, 19.3397)
  line L674 (-33, 19.3397) -> (-33, 36.6603)
  line L675 (-33, 19.3397) -> (-33, 36.6603)
  line L676 (-48, 45.3205) -> (-63, 36.6603)
  line L677 (-33, 36.6603) -> (-48, 45.3205)
  line L678 (-16, 45.3205) -> (-31, 36.6603)
  line L679 (-1, 36.6603) -> (-16, 45.3205)
  line L680 (16, 45.3205) -> (1, 36.6603)
  line L681 (31, 36.6603) -> (16, 45.3205)
  line L682 (48, 45.3205) -> (33, 36.6603)
  line L683 (63, 36.6603) -> (48, 45.3205)
  line L684 (48, 10.6795) -> (63, 19.3397)
  line L685 (33, 19.3397) -> (48, 10.6795)
  line L686 (16, 10.6795) -> (31, 19.3397)
  line L687 (1, 19.3397) -> (16, 10.6795)
  line L688 (-16, 10.6795) -> (-1, 19.3397)
  line L689 (-31, 19.3397) -> (-16, 10.6795)
  line L690 (-48, 10.6795) -> (-33, 19.3397)
  line L691 (-63, 19.3397) -> (-48, 10.6795)
  line L692 (-15, 8.6603) -> (-15, -8.6603)
  line L693 (17, 8.6603) -> (17, -8.6603)
  line L694 (49, 8.6603) -> (49, -8.6603)
  line L695 (-64, -17.3205) -> (-49, -8.6603)
  line L696 (17, 8.6603) -> (17, -8.6603)
  line L697 (-15, 8.6603) -> (-15, -8.6603)
  line L698 (-49, -8.6603) -> (-49, 8.6603)
  line L699 (-64, -17.3205) -> (-49, -8.6603)
  line L700 (47, -8.6603) -> (47, 8.6603)
  line L701 (-47, 8.6603) -> (-47, -8.6603)
  line L702 (-17, -8.6603) -> (-17, 8.6603)
  line L703 (15, -8.6603) -> (15, 8.6603)
  line L704 (-79, -8.6603) -> (-64, -17.3205)
  line L705 (-47, 8.6603) -> (-47, -8.6603)
  line L706 (49, 8.6603) -> (49, -8.6603)
  line L707 (-79, -8.6603) -> (-64, -17.3205)
  line L708 (-64, -17.3205) -> (-49, -8.6603)
  line L709 (-64, -17.3205) -> (-49, -8.6603)
  line L710 (-49, -8.6603) -> (-49, 8.6603)
  line L711 (-79, 8.6603) -> (-79, -8.6603)
  line L712 (15, -8.6603) -> (15, 8.6603)
  line L713 (79, -8.6603) -> (79, 8.6603)
  line L714 (-17, -8.6603) -> (-17, 8.6603)
  line L715 (63, -19.3397) -> (48, -10.6795)
  line L716 (31, -19.3397) -> (16, -10.6795)
  line L717 (32, -17.3205) -> (47, -8.6603)
  line L718 (31, -19.3397) -> (16, -10.6795)
  line L719 (16, -10.6795) -> (1, -19.3397)
  line L720 (16, -10.6795) -> (1, -19.3397)
  line L721 (16, -10.6795) -> (1, -19.3397)
  line L722 (16, -10.6795) -> (1, -19.3397)
  line L723 (31, -19.3397) -> (16, -10.6795)
  line L724 (16, -10.6795) -> (1, -19.3397)
  line L725 (16, -10.6795) -> (1, -19.3397)
  line L726 (64, -17.3205) -> (79, -8.6603)
  line L727 (16, -10.6795) -> (1, -19.3397)
  line L728 (49, -8.6603) -> (64, -17.3205)
  line L729 (31, -19.3397) -> (16, -10.6795)
  line L730 (31, -19.3397) -> (16, -10.6795)
  line L731 (16, -10.6795) -> (1, -19.3397)
  line L732 (32, -17.3205) -> (47, -8.6603)
  line L733 (31, -19.3397) -> (16, -10.6795)
  line L734 (16, -10.6795) -> (1, -19.3397)
  line L735 (16, -10.6795) -> (1, -19.3397)
  line L736 (31, -19.3397) -> (16, -10.6795)
  line L737 (48, -10.6795) -> (33, -19.3397)
  line L738 (31, -19.3397) -> (16, -10.6795)
  line L739 (-1, -19.3397) -> (-16, -10.6795)
  line L740 (63, -19.3397) -> (48, -10.6795)
  line L741 (16, -10.6795) -> (1, -19.3397)
  line L742 (63, -19.3397) -> (48, -10.6795)
  line L743 (-1, -19.3397) -> (-16, -10.6795)
  line L744 (16, -10.6795) -> (1, -19.3397)
  line L745 (-1, -19.3397) -> (-16, -10.6795)
  line L746 (-1, -19.3397) -> (-16, -10.6795)
  line L747 (16, -10.6795) -> (1, -19.3397)
  line L748 (49, -8.6603) -> (64, -17.3205)
  line L749 (-15, -8.6603) -> (0, -17.3205)
  line L750 (32, -17.3205) -> (47, -8.6603)
  line L751 (-47, -8.6603) -> (-32, -17.3205)
  line L752 (-1, -19.3397) -> (-16, -10.6795)
  line L753 (48, -10.6795) -> (33, -19.3397)
  line L754 (16, -10.6795) -> (1, -19.3397)
  line L755 (31, -19.3397) -> (16, -10.6795)
  line L756 (-15, -8.6603) -> (0, -17.3205)
  line L757 (-33, -19.3397) -> (-48, -10.6795)
  line L758 (-47, -8.6603) -> (-32, -17.3205)
  line L759 (15, 8.6603) -> (0, 17.3205)
  line L760 (31, -19.3397) -> (16, -10.6795)
  line L761 (48, -10.6795) -> (33, -19.3397)
  line L762 (-1, -19.3397) -> (-16, -10.6795)
  line L763 (-1, -19.3397) -> (-16, -10.6795)
  line L764 (-47, -8.6603) -> (-32, -17.3205)
  line L765 (64, -17.3205) -> (79, -8.6603)
  line L766 (-32, 17.3205) -> (-47, 8.6603)
  line L767 (31, -19.3397) -> (16, -10.6795)
  line L768 (49, -8.6603) -> (64, -17.3205)
  line L769 (16, -10.6795) -> (1, -19.3397)
  line L770 (-17, 8.6603) -> (-32, 17.3205)
  line L771 (64, -17.3205) -> (79, -8.6603)
  line L772 (48, -10.6795) -> (33, -19.3397)
  line L773 (32, -17.3205) -> (47, -8.6603)
  line L774 (-33, -19.3397) -> (-48, -10.6795)
  line L775 (-47, -8.6603) -> (-32, -17.3205)
  line L776 (-1, -19.3397) -> (-16, -10.6795)
  line L777 (31, -19.3397) -> (16, -10.6795)
  line L778 (63, -19.3397) -> (48, -10.6795)
  line L779 (-1, -19.3397) -> (-16, -10.6795)
  line L780 (-1, -19.3397) -> (-16, -10.6795)
  line L781 (-48, -10.6795) -> (-63, -19.3397)
  line L782 (49, -8.6603) -> (64, -17.3205)
  line L783 (64, -17.3205) -> (79, -8.6603)
  line L784 (31, -19.3397) -> (16, -10.6795)
  line L785 (31, -19.3397) -> (16, -10.6795)
  line L786 (31, -19.3397) -> (16, -10.6795)
  line L787 (-15, -8.6603) -> (0, -17.3205)
  line L788 (16, -10.6795) -> (1, -19.3397)
  line L789 (15, 8.6603) -> (0, 17.3205)
  line L790 (31, -19.3397) -> (16, -10.6795)
  line L791 (-15, -8.6603) -> (0, -17.3205)
  line L792 (0, -17.3205) -> (15, -8.6603)
  line L793 (-16, -10.6795) -> (-31, -19.3397)
  line L794 (0, 17.3205) -> (-15, 8.6603)
  line L795 (-64, 17.3205) -> (-79, 8.6603)
  line L796 (-16, -10.6795) -> (-31, -19.3397)
  line L797 (47, 8.6603) -> (32, 17.3205)
  line L798 (0, -17.3205) -> (15, -8.6603)
  line L799 (-79, -8.6603) -> (-64, -17.3205)
  line L800 (-16, -10.6795) -> (-31, -19.3397)
  line L801 (-79, 8.6603) -> (-79, -8.6603)
  line L802 (47, -8.6603) -> (47, 8.6603)
  line L803 (-16, -10.6795) -> (-31, -19.3397)
  line L804 (-16, -10.6795) -> (-31, -19.3397)
  line L805 (-16, -10.6795) -> (-31, -19.3397)
  line L806 (-16, -10.6795) -> (-31, -19.3397)
  line L807 (-32, -17.3205) -> (-17, -8.6603)
  line L808 (-49, 8.6603) -> (-64, 17.3205)
  line L809 (32, 17.3205) -> (17, 8.6603)
  line L810 (0, -17.3205) -> (15, -8.6603)
  line L811 (0, 17.3205) -> (-15, 8.6603)
  line L812 (-16, 10.6795) -> (-1, 19.3397)
  line L813 (-16, -10.6795) -> (-31, -19.3397)
  line L814 (-16, -10.6795) -> (-31, -19.3397)
  line L815 (-32, -17.3205) -> (-17, -8.6603)
  line L816 (79, -8.6603) -> (79, 8.6603)
  line L817 (-16, -10.6795) -> (-31, -19.3397)
  line L818 (-16, -10.6795) -> (-31, -19.3397)
  line L819 (-48, 10.6795) -> (-33, 19.3397)
  line L820 (0, -17.3205) -> (15, -8.6603)
  line L821 (-16, -10.6795) -> (-31, -19.3397)
  line L822 (-79, -8.6603) -> (-64, -17.3205)
  line L823 (16, 10.6795) -> (31, 19.3397)
  line L824 (-32, -17.3205) -> (-17, -8.6603)
  line L825 (32, 17.3205) -> (17, 8.6603)
  line L826 (-49, 8.6603) -> (-64, 17.3205)
  line L827 (-64, 17.3205) -> (-79, 8.6603)
  line L828 (79, 8.6603) -> (64, 17.3205)
  line L829 (17, -8.6603) -> (32, -17.3205)
  line L830 (-1, -19.3397) -> (-16, -10.6795)
  line L831 (-1, -19.3397) -> (-16, -10.6795)
  line L832 (-63, 19.3397) -> (-48, 10.6795)
  line L833 (-48, -10.6795) -> (-63, -19.3397)
  line L834 (-33, -19.3397) -> (-48, -10.6795)
  line L835 (-48, -10.6795) -> (-63, -19.3397)
  line L836 (47, 8.6603) -> (32, 17.3205)
  line L837 (-48, -10.6795) -> (-63, -19.3397)
  line L838 (-1, -19.3397) -> (-16, -10.6795)
  line L839 (-33, -19.3397) -> (-48, -10.6795)
  line L840 (-48, -10.6795) -> (-63, -19.3397)
  line L841 (-48, -10.6795) -> (-63, -19.3397)
  line L842 (17, -8.6603) -> (32, -17.3205)
  line L843 (-33, -19.3397) -> (-48, -10.6795)
  line L844 (-48, -10.6795) -> (-63, -19.3397)
  line L845 (-33, -19.3397) -> (-48, -10.6795)
  line L846 (-33, -19.3397) -> (-48, -10.6795)
  line L847 (-33, -19.3397) -> (-48, -10.6795)
  line L848 (-1, -19.3397) -> (-16, -10.6795)
  line L849 (-17, 8.6603) -> (-32, 17.3205)
  line L850 (-48, -10.6795) -> (-63, -19.3397)
  line L851 (-31, 19.3397) -> (-16, 10.6795)
  line L852 (-48, -10.6795) -> (-63, -19.3397)
  line L853 (-48, -10.6795) -> (-63, -19.3397)
  line L854 (64, 17.3205) -> (49, 8.6603)
  line L855 (79, 8.6603) -> (64, 17.3205)
  line L856 (-33, -19.3397) -> (-48, -10.6795)
  line L857 (33, 19.3397) -> (48, 10.6795)
  line L858 (-48, -10.6795) -> (-63, -19.3397)
  line L859 (64, 17.3205) -> (49, 8.6603)
  line L860 (48, 10.6795) -> (63, 19.3397)
  line L861 (-48, -10.6795) -> (-63, -19.3397)
  line L862 (-48, -10.6795) -> (-63, -19.3397)
  line L863 (-33, -19.3397) -> (-48, -10.6795)
  line L864 (-16, -10.6795) -> (-31, -19.3397)
  line L865 (-1, -19.3397) -> (-16, -10.6795)
  line L866 (-48, -10.6795) -> (-63, -19.3397)
  line L867 (-16, -10.6795) -> (-31, -19.3397)
  line L868 (-33, -19.3397) -> (-48, -10.6795)
  line L869 (-33, -19.3397) -> (-48, -10.6795)
  line L870 (-33, -19.3397) -> (-48, -10.6795)
  line L871 (-33, -19.3397) -> (-48, -10.6795)
  line L872 (-33, -19.3397) -> (-48, -10.6795)
  line L873 (-16, -10.6795) -> (-31, -19.3397)
  line L874 (-32, 17.3205) -> (-47, 8.6603)
  line L875 (17, -8.6603) -> (32, -17.3205)
  line L876 (1, 19.3397) -> (16, 10.6795)
  line L877 (-32, -17.3205) -> (-17, -8.6603)
  line L878 (-16, -10.6795) -> (-31, -19.3397)
  line L879 (-48, -10.6795) -> (-63, -19.3397)
  line L880 (-33, -19.3397) -> (-48, -10.6795)
  line L881 (17, -8.6603) -> (32, -17.3205)
  line L882 (-48, -10.6795) -> (-63, -19.3397)
  line L883 (-1, -19.3397) -> (-16, -10.6795)
  line L884 (-17, -8.6603) -> (-17, 8.6603)
  line L885 (79, -8.6603) -> (79, 8.6603)
  line L886 (-63, -19.3397) -> (-63, -36.6603)
  line L887 (-63, -19.3397) -> (-63, -36.6603)
  line L888 (-79, -8.6603) -> (-64, -17.3205)
  line L889 (-79, -8.6603) -> (-64, -17.3205)
  line L890 (-64, -17.3205) -> (-49, -8.6603)
  line L891 (-64, -17.3205) -> (-49, -8.6603)
  line L892 (-64, -17.3205) -> (-49, -8.6603)
  line L893 (-64, -17.3205) -> (-49, -8.6603)
  line L894 (-63, -19.3397) -> (-63, -36.6603)
  line L895 (-63, -19.3397) -> (-63, -36.6603)
  line L896 (-63, -19.3397) -> (-63, -36.6603)
  line L897 (-63, -19.3397) -> (-63, -36.6603)
  line L898 (-63, -19.3397) -> (-63, -36.6603)
  line L899 (-63, -19.3397) -> (-63, -36.6603)
  line L900 (-63, -19.3397) -> (-63, -36.6603)
  line L901 (-63, -19.3397) -> (-63, -36.6603)
  line L902 (-63, -19.3397) -> (-63, -36.6603)
  line L903 (-63, -19.3397) -> (-63, -36.6603)
  line L904 (-63, -19.3397) -> (-63, -36.6603)
  line L905 (-63, -19.3397) -> (-63, -36.6603)
  line L906 (-63, -19.3397) -> (-63, -36.6603)
  line L907 (-63, -19.3397) -> (-63, -36.6603)
  line L908 (-79, 8.6603) -> (-79, -8.6603)
  line L909 (47, -8.6603) -> (47, 8.6603)
  line L910 (17, 8.6603) -> (17, -8.6603)
  line L911 (49, -8.6603) -> (64, -17.3205)
  line L912 (16, -10.6795) -> (1, -19.3397)
  line L913 (49, -8.6603) -> (64, -17.3205)
  line L914 (16, -10.6795) -> (1, -19.3397)
  line L915 (16, -10.6795) -> (1, -19.3397)
  line L916 (-48, -10.6795) -> (-63, -19.3397)
  line L917 (32, -17.3205) -> (47, -8.6603)
  line L918 (-1, -19.3397) -> (-16, -10.6795)
  line L919 (63, -19.3397) -> (48, -10.6795)
  line L920 (-1, -19.3397) -> (-16, -10.6795)
  line L921 (31, -19.3397) -> (16, -10.6795)
  line L922 (-33, -19.3397) -> (-48, -10.6795)
  line L923 (-1, -19.3397) -> (-16, -10.6795)
  line L924 (-48, -10.6795) -> (-63, -19.3397)
  line L925 (-33, -19.3397) -> (-48, -10.6795)
  line L926 (-48, -10.6795) -> (-63, -19.3397)
  line L927 (-47, -8.6603) -> (-32, -17.3205)
  line L928 (-1, -19.3397) -> (-16, -10.6795)
  line L929 (64, -17.3205) -> (79, -8.6603)
  line L930 (31, -19.3397) -> (16, -10.6795)
  line L931 (49, -8.6603) -> (64, -17.3205)
  line L932 (-33, -19.3397) -> (-48, -10.6795)
  line L933 (16, -10.6795) -> (1, -19.3397)
  line L934 (31, -19.3397) -> (16, -10.6795)
  line L935 (32, -17.3205) -> (47, -8.6603)
  line L936 (-33, -19.3397) -> (-48, -10.6795)
  line L937 (63, -19.3397) -> (48, -10.6795)
  line L938 (31, -19.3397) -> (16, -10.6795)
  line L939 (-47, -8.6603) -> (-32, -17.3205)
  line L940 (-48, -10.6795) -> (-63, -19.3397)
  line L941 (16, -10.6795) -> (1, -19.3397)
  line L942 (-1, -19.3397) -> (-16, -10.6795)
  line L943 (-1, -19.3397) -> (-16, -10.6795)
  line L944 (64, -17.3205) -> (79, -8.6603)
  line L945 (64, -17.3205) -> (79, -8.6603)
  line L946 (-33, -19.3397) -> (-48, -10.6795)
  line L947 (32, -17.3205) -> (47, -8.6603)
  line L948 (-48, -10.6795) -> (-63, -19.3397)
  line L949 (32, -17.3205) -> (47, -8.6603)
  line L950 (32, -17.3205) -> (47, -8.6603)
  line L951 (49, -8.6603) -> (64, -17.3205)
  line L952 (-47, -8.6603) -> (-32, -17.3205)
  line L953 (-47, -8.6603) -> (-32, -17.3205)
  line L954 (-1, -19.3397) -> (-16, -10.6795)
  line L955 (16, -10.6795) -> (1, -19.3397)
  line L956 (31, -19.3397) -> (16, -10.6795)
  line L957 (-1, -19.3397) -> (-16, -10.6795)
  line L958 (-1, -36.6603) -> (-1, -19.3397)
  line L959 (32, -17.3205) -> (47, -8.6603)
  line L960 (-47, -8.6603) -> (-32, -17.3205)
  line L961 (64, -17.3205) -> (79, -8.6603)
  line L962 (-1, -19.3397) -> (-16, -10.6795)
  line L963 (-47, -8.6603) -> (-32, -17.3205)
  line L964 (16, -10.6795) -> (1, -19.3397)
  line L965 (-48, -10.6795) -> (-63, -19.3397)
  line L966 (16, -10.6795) -> (1, -19.3397)
  line L967 (32, -17.3205) -> (47, -8.6603)
  line L968 (32, -17.3205) -> (47, -8.6603)
  line L969 (49, -8.6603) -> (64, -17.3205)
  line L970 (31, -19.3397) -> (16, -10.6795)
  line L971 (-15, -8.6603) -> (0, -17.3205)
  line L972 (49, -8.6603) -> (64, -17.3205)
  line L973 (-47, -8.6603) -> (-32, -17.3205)
  line L974 (16, -10.6795) -> (1, -19.3397)
  line L975 (-33, -19.3397) -> (-48, -10.6795)
  line L976 (-15, -8.6603) -> (0, -17.3205)
  line L977 (-48, -10.6795) -> (-63, -19.3397)
  line L978 (-48, -10.6795) -> (-63, -19.3397)
  line L979 (-1, -19.3397) -> (-16, -10.6795)
  line L980 (-15, -8.6603) -> (0, -17.3205)
  line L981 (16, -10.6795) -> (1, -19.3397)
  line L982 (-33, -19.3397) -> (-48, -10.6795)
  line L983 (-48, -10.6795) -> (-63, -19.3397)
  line L984 (31, -19.3397) -> (16, -10.6795)
  line L985 (-15, -8.6603) -> (0, -17.3205)
  line L986 (-48, -10.6795) -> (-63, -19.3397)
  line L987 (-1, -19.3397) -> (-16, -10.6795)
  line L988 (16, -10.6795) -> (1, -19.3397)
  line L989 (-1, -19.3397) -> (-16, -10.6795)
  line L990 (-33, -19.3397) -> (-48, -10.6795)
  line L991 (-33, -19.3397) -> (-48, -10.6795)
  line L992 (31, -19.3397) -> (16, -10.6795)
  line L993 (-48, -10.6795) -> (-63, -19.3397)
  line L994 (64, -17.3205) -> (79, -8.6603)
  line L995 (-1, -19.3397) -> (-16, -10.6795)
  line L996 (-33, -19.3397) -> (-48, -10.6795)
  line L997 (-48, -10.6795) -> (-63, -19.3397)
  line L998 (16, -10.6795) -> (1, -19.3397)
  line L999 (31, -19.3397) -> (16, -10.6795)
  line L1000 (-33, -19.3397) -> (-48, -10.6795)
  line L1001 (-48, -10.6795) -> (-63, -19.3397)
  line L1002 (49, -8.6603) -> (64, -17.3205)
  line L1003 (16, -10.6795) -> (1, -19.3397)
  line L1004 (16, -10.6795) -> (1, -19.3397)
  line L1005 (-33, -19.3397) -> (-48, -10.6795)
  line L1006 (-1, -19.3397) -> (-16, -10.6795)
  line L1007 (-1, -19.3397) -> (-16, -10.6795)
  line L1008 (49, -8.6603) -> (64, -17.3205)
  line L1009 (16, -10.6795) -> (1, -19.3397)
  line L1010 (16, -10.6795) -> (1, -19.3397)
  line L1011 (-1, -19.3397) -> (-16, -10.6795)
  line L1012 (64, -17.3205) -> (79, -8.6603)
  line L1013 (-33, -19.3397) -> (-48, -10.6795)
  line L1014 (64, -17.3205) -> (79, -8.6603)
  line L1015 (-1, -19.3397) -> (-16, -10.6795)
  line L1016 (-15, -8.6603) -> (0, -17.3205)
  line L1017 (16, -10.6795) -> (1, -19.3397)
  line L1018 (16, -10.6795) -> (1, -19.3397)
  line L1019 (64, -17.3205) -> (79, -8.6603)
  line L1020 (-1, -19.3397) -> (-16, -10.6795)
  line L1021 (-48, -10.6795) -> (-63, -19.3397)
  line L1022 (16, -10.6795) -> (1, -19.3397)
  line L1023 (16, -10.6795) -> (1, -19.3397)
  line L1024 (-15, -8.6603) -> (0, -17.3205)
  line L1025 (-33, -19.3397) -> (-48, -10.6795)
  line L1026 (16, -10.6795) -> (1, -19.3397)
  line L1027 (-15, -8.6603) -> (0, -17.3205)
  line L1028 (16, -10.6795) -> (1, -19.3397)
  line L1029 (-48, -10.6795) -> (-63, -19.3397)
  line L1030 (-1, -19.3397) -> (-16, -10.6795)
  line L1031 (31, -19.3397) -> (16, -10.6795)
  line L1032 (-48, -10.6795) -> (-63, -19.3397)
  line L1033 (-48, -10.6795) -> (-63, -19.3397)
  line L1034 (-15, -8.6603) -> (0, -17.3205)
  line L1035 (31, -19.3397) -> (16, -10.6795)
  line L1036 (-48, -10.6795) -> (-63, -19.3397)
  line L1037 (31, -19.3397) -> (16, -10.6795)
  line L1038 (31, -19.3397) -> (16, -10.6795)
  line L1039 (31, -19.3397) -> (16, -10.6795)
  line L1040 (-33, -19.3397) -> (-48, -10.6795)
  line L1041 (-48, -10.6795) -> (-63, -19.3397)
  line L1042 (31, -19.3397) -> (16, -10.6795)
  line L1043 (-48, -10.6795) -> (-63, -19.3397)
  line L1044 (16, -10.6795) -> (1, -19.3397)
  line L1045 (-48, -10.6795) -> (-63, -19.3397)
  line L1046 (-33, -19.3397) -> (-48, -10.6795)
  line L1047 (31, -19.3397) -> (16, -10.6795)
  line L1048 (-33, -19.3397) -> (-48, -10.6795)
  line L1049 (31, -19.3397) -> (16, -10.6795)
  line L1050 (16, -10.6795) -> (1, -19.3397)
  line L1051 (31, -19.3397) -> (16, -10.6795)
  line L1052 (31, -19.3397) -> (16, -10.6795)
  line L1053 (16, -10.6795) -> (1, -19.3397)
  line L1054 (16, -10.6795) -> (1, -19.3397)
  line L1055 (16, -10.6795) -> (1, -19.3397)
  line L1056 (-33, -19.3397) -> (-48, -10.6795)
  line L1057 (16, -10.6795) -> (1, -19.3397)
  line L1058 (31, -19.3397) -> (16, -10.6795)
  line L1059 (31, -19.3397) -> (16, -10.6795)
  line L1060 (-33, -19.3397) -> (-48, -10.6795)
  line L1061 (-33, -19.3397) -> (-48, -10.6795)
  line L1062 (-48, -10.6795) -> (-63, -19.3397)
  line L1063 (31, -19.3397) -> (16, -10.6795)
  line L1064 (-33, -19.3397) -> (-48, -10.6795)
  line L1065 (-33, -19.3397) -> (-48, -10.6795)
  line L1066 (16, -10.6795) -> (1, -19.3397)
  line L1067 (31, -19.3397) -> (16, -10.6795)
  line L1068 (63, -19.3397) -> (48, -10.6795)
  line L1069 (17, -8.6603) -> (32, -17.3205)
  line L1070 (-47, -8.6603) -> (-32, -17.3205)
  line L1071 (-33, -19.3397) -> (-48, -10.6795)
  line L1072 (-1, -19.3397) -> (-16, -10.6795)
  line L1073 (-48, -10.6795) -> (-63, -19.3397)
  line L1074 (48, -10.6795) -> (33, -19.3397)
  line L1075 (48, -10.6795) -> (33, -19.3397)
  line L1076 (16, -10.6795) -> (1, -19.3397)
  line L1077 (-1, -19.3397) -> (-16, -10.6795)
  line L1078 (-33, -19.3397) -> (-48, -10.6795)
  line L1079 (31, -19.3397) -> (16, -10.6795)
  line L1080 (-33, -19.3397) -> (-48, -10.6795)
  line L1081 (-48, -10.6795) -> (-63, -19.3397)
  line L1082 (-33, -36.6603) -> (-33, -19.3397)
  line L1083 (48, -10.6795) -> (33, -19.3397)
  line L1084 (-1, -36.6603) -> (-1, -19.3397)
  line L1085 (-48, -10.6795) -> (-63, -19.3397)
  line L1086 (-1, -19.3397) -> (-16, -10.6795)
  line L1087 (-1, -19.3397) -> (-16, -10.6795)
  line L1088 (31, -19.3397) -> (16, -10.6795)
  line L1089 (48, -10.6795) -> (33, -19.3397)
  line L1090 (-1, -19.3397) -> (-16, -10.6795)
  line L1091 (31, -19.3397) -> (16, -10.6795)
  line L1092 (63, -19.3397) -> (48, -10.6795)
  line L1093 (16, -10.6795) -> (1, -19.3397)
  line L1094 (-33, -19.3397) -> (-48, -10.6795)
  line L1095 (-1, -36.6603) -> (-1, -19.3397)
  line L1096 (-31, -19.3397) -> (-31, -36.6603)
  line L1097 (31, -19.3397) -> (16, -10.6795)
  line L1098 (63, -19.3397) -> (48, -10.6795)